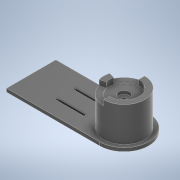
# Autodesk Inventor part: Base
Saved by Autodesk Inventor 2022.3 (Build 263350000, 350)
## iProperties
Created: 2022-05-27
Part Number: Base
Material: PC/ABS Plastic
Document SubType Name: Modeling
Designer: Mlees
Density: 0.357273 g/cm^3
Appearance: Smooth - White
Author: Mlees
Autodesk Inventor part; units mm, degrees
ref_plane "YZ Plane" through (0, 0, 0) normal (1, 0, 0) x (0, 1, 0)
ref_plane "XZ Plane" through (0, 0, 0) normal (0, 1, 0) x (-1, 0, 0)
ref_plane "XY Plane" through (0, 0, 0) normal (0, 0, 1) x (1, 0, 0)
sketch "Sketch1" plane through (0, 0, 0) normal (0, 1, 0) x (-1, 0, 0)
  line L0 (-100, 300) -> (100, 300)
  line L1 (100, 300) -> (100, -100)
  line L2 (100, -100) -> (-100, -100)
  line L3 (-100, -100) -> (-100, 300)
  point P0 (0, 0)
  dimension "d4" = 200
  dimension "d5" = 400
  constraints: 8 end point, 2 parallel, 1 horizontal, 1 perpendicular
  measures "d4" distance of L1.end L2.end
  measures "d5" distance of L0.end L1.end
extrude "Extrusion1" add sketch "Sketch1" along normal blind 5
sketch "Sketch2" plane through (0, 5, 0) normal (0, 1, 0) x (1, 0, 0)
  circle A0 centre (0, 0) radius 3
  circle A1 centre (0, 0) radius 30
  dimension "d10" = 6
  dimension "d11" = 60
  constraints: 2 centre point, 2 coincident
  measures "d10" diameter of A0
  measures "d11" diameter of A1
extrude "Extrusion2" add sketch "Sketch2" along normal blind 41.5
sketch "Sketch3" plane through (0, 46.5, 0) normal (0, 1, 0) x (1, 0, 0)
  circle A0 centre (0, 0) radius 3 projected
  circle A1 centre (0, 0) radius 30
  circle A2 centre (0, 0) radius 21.5
  circle A3 centre (0, 0) radius 3
  dimension "d14" = 43
  dimension "d15" = 6
  constraints: 3 centre point, 3 coincident
  measures "d14" diameter of A2
  measures "d15" diameter of A3
extrude "Extrusion3" add sketch "Sketch3" along normal blind 1 contours A1
sketch "Sketch4" plane through (0, 47.5, 0) normal (0, 1, 0) x (1, 0, 0)
  circle A0 centre (0, 0) radius 21.5 projected
  line L0 (-21.5, 0) -> (-30, 0)
  circle A1 centre (0, 0) radius 30 projected
  line L1 (21.633, 0) -> (30.1771, 0)
  circle A2 centre (0, 0) radius 3 projected
  arc A3 (21.633, 0) -> (-21.633, 0) centre (0, 0) ccw
  point P0 (30, 0)
  constraints: 4 end point, 3 point on line, 2 point on circle, 1 centre point, 1 coincident, 1 horizontal, 1 horizontal alignment, 3 other
extrude "Extrusion4" add sketch "Sketch4" along normal blind 15 contours L0 A1 L1 A3 picked at (-26.7109, 4.1189)
sketch "Sketch5" plane through (0, 5, 0) normal (0, 1, 0) x (1, 0, 0)
  line L0 (-13, 0) -> (13, 0)
  arc A0 (-11.5, -45) -> (-14.5, -45) centre (-13, -45) ccw
  line L1 (-14.5, -45) -> (-14.5, -85)
  arc A1 (-14.5, -85) -> (-11.5, -85) centre (-13, -85) ccw
  line L2 (-11.5, -45) -> (-11.5, -85)
  line L3 (0, 0) -> (0, -51.7204)
  arc A2 (14.5, -45) -> (11.5, -45) centre (13, -45) ccw
  line L4 (14.5, -45) -> (14.5, -85)
  arc A3 (11.5, -85) -> (14.5, -85) centre (13, -85) ccw
  line L5 (11.5, -45) -> (11.5, -85)
  dimension "d20" = 13
  dimension "d21" = 26
  dimension "d22" = 45
  dimension "d24" = 40
  constraints: 12 end point, 8 point on circle, 5 symmetric about line, 4 centre point, 2 tangent, 2 vertical, 2 other
  measures "d20" distance of L3.start L0.start
  measures "d21" distance of L0.start L0.end
  measures "d22" distance of L0.end A2.centre
  measures "d24" distance of L1.start L1.end
extrude "Extrusion5" cut sketch "Sketch5" against normal through all
fillet "Fillet1" radius 2 8 edges at (13, 0, 43.5) (11.5, 0, 65) (13, 0, 86.5) (14.5, 0, 65) (-13, 0, 43.5) (-14.5, 0, 65) (-13, 0, 86.5) (-11.5, 0, 65) inverted yes
sketch "Sketch6" plane through (0, 47.5, 0) normal (0, 1, 0) x (1, 0, 0)
  circle A0 centre (0, 0) radius 3 projected
  circle A1 centre (0, 0) radius 30
  circle A2 centre (0, 0) radius 21.5
  circle A3 centre (0, 0) radius 30 projected
  line L0 (0, 0) -> (30, 0) construction
  line L1 (0, 0) -> (30, 0) construction
  line L2 (-5.5646, -20.7674) -> (-7.7646, -28.9778)
  line L3 (5.5646, -20.7674) -> (7.7646, -28.9778)
  constraints: 8 end point, 4 point on circle, 2 centre point, 2 coincident, 2 horizontal
extrude "Extrusion6" add sketch "Sketch6" along normal up to surface (15 mm away) contours L2 A2 L3 A1 picked at (5.3146, -26.5437)
sketch "Sketch7" plane through (0, 5, 0) normal (0, 1, 0) x (1, 0, 0)
  circle A0 centre (0, 0) radius 3 projected
  line L0 (-50, 0) -> (-50, 50)
  line L1 (-50, 50) -> (50, 50)
  line L2 (50, 50) -> (50, -150)
  line L3 (50, -150) -> (-50, -150)
  line L4 (-50, -150) -> (-50, 0)
  line L5 (-100, 100) -> (-100, -300) projected
  line L6 (-100, -300) -> (100, -300)
  line L7 (100, -300) -> (100, 100)
  line L8 (100, 100) -> (-100, 100)
  line L9 (-100, 100) -> (-100, -300)
  dimension "d32" = 50
  dimension "d33" = 50
  dimension "d34" = 100
  dimension "d35" = 200
  constraints: 18 end point, 4 perpendicular, 2 parallel, 1 collinear, 1 horizontal, 1 point on line, 1 vertical
  measures "d32" distance of A0.centre L0.start
  measures "d33" distance of L0.start L0.end
  measures "d34" distance of L0.end L1.end
  measures "d35" distance of L1.end L2.end
extrude "Extrusion7" cut sketch "Sketch7" against normal through all contours L8 L7 L6 L5
sketch "Sketch8" plane through (0, 62.5, 0) normal (0, 1, 0) x (1, 0, 0)
  circle A0 centre (0, 0) radius 3 projected
  arc A1 (-7.7646, -28.9778) -> (7.7646, -28.9778) centre (0, 0) ccw projected
  circle A2 centre (0, 0) radius 30
  line L0 (-7.7646, -28.9778) -> (-5.5646, -20.7674) projected
  circle A3 centre (0, 0) radius 21.5
  line L1 (-5.5646, -20.7674) -> (-7.7646, -28.9778)
  line L2 (5.5646, -20.7674) -> (7.7646, -28.9778) projected
  line L3 (5.5646, -20.7674) -> (7.7646, -28.9778)
  arc A4 (21.633, 0) -> (-21.633, 0) centre (0, 0) ccw projected
  line L4 (-21.633, 0) -> (-30, 0) projected
  line L5 (-21.633, 0) -> (-30, 0)
  line L6 (21.633, 0) -> (30, 0) projected
  arc A5 (30, 0) -> (-30, 0) centre (0, 0) ccw projected
  line L7 (21.633, 0) -> (30, 0)
  constraints: 8 end point, 2 centre point, 2 coincident, 2 collinear, 2 horizontal, 2 point on circle
extrude "Extrusion8" cut sketch "Sketch8" against normal blind 7 contours L0 A3 L2 A1 | A2 L6 A4 L4
sketch "Sketch10" plane through (0, 46.5, 0) normal (0, 1, 0) x (1, 0, 0)
  circle A0 centre (0, 0) radius 8.125
  constraints: 1 centre point, 1 coincident
extrude "Extrusion10" cut sketch "Sketch10" against normal blind 5
sketch "Sketch11" plane through (-50, 5, 150) normal (0, 0, 1) x (1, 0, 0)
  line L0 (100, 0) -> (100, -5) projected
  line L1 (0, -5) -> (100, -5)
  line L2 (100, -5) -> (100, 0)
  line L3 (100, 0) -> (0, 0)
  line L4 (0, 0) -> (0, -5)
  point P0 (50, -5)
  constraints: 8 end point, 2 parallel, 1 horizontal, 1 perpendicular
extrude "Extrusion11" cut sketch "Sketch11" against normal blind 14
sketch "Sketch12" plane through (0, 5, 0) normal (0, 1, 0) x (1, 0, 0)
  arc A0 (36, 0) -> (-36, 0) centre (0, 0) ccw
  line L0 (36, 0) -> (36, -136)
  line L1 (50, -136) -> (-50, -136) projected
  line L2 (50, 50) -> (50, -136) projected
  line L3 (36, -136) -> (50, -136)
  line L4 (50, -136) -> (50, 50)
  line L5 (50, 50) -> (-50, 50)
  line L6 (-50, -136) -> (-50, 50) projected
  line L7 (-50, 50) -> (-50, -136)
  line L8 (-50, -136) -> (-36, -136)
  line L9 (-36, -136) -> (-36, 0)
  dimension "d47" = 72
  constraints: 14 end point, 2 collinear, 2 perpendicular, 2 point on circle, 2 point on line, 1 centre point, 1 coincident, 1 tangent, 1 vertical
  measures "d47" diameter of A0
extrude "Extrusion12" cut sketch "Sketch12" against normal through all contours A0 L9 L1 L6 L5 L2 L0
sketch "Sketch13" plane through (0, 0, 0) normal (0, -1, 0) x (1, 0, 0)
  circle A0 centre (0, 0) radius 3 projected
  line L0 (0, -12.5) -> (12.5, -12.5)
  line L1 (12.5, -12.5) -> (-12.5, -12.5)
  line L2 (-12.5, -12.5) -> (-12.5, 12.5)
  line L3 (-12.5, 12.5) -> (12.5, 12.5)
  line L4 (12.5, 12.5) -> (12.5, -12.5)
  dimension "d50" = 12.5
  dimension "d51" = 12.5
  dimension "d52" = 25
  dimension "d53" = 25
  constraints: 10 end point, 2 parallel, 1 horizontal, 1 perpendicular
  measures "d50" distance of A0.centre L0.start
  measures "d51" distance of L0.start L0.end
  measures "d52" distance of L2.end L3.end
  measures "d53" distance of L1.end L2.end
extrude "Extrusion13" cut sketch "Sketch13" against normal blind 12.5 contours A0 | L1 L2 L3 L4 L0
sketch "Sketch14" plane through (0, 0, 0) normal (0, -1, 0) x (1, 0, 0)
  line L0 (-12.5, 12.5) -> (12.5, 12.5) projected
  line L1 (12.5, 12.5) -> (-12.5, 12.5)
  line L2 (-12.5, 12.5) -> (-12.5, 18.5)
  line L3 (-12.5, 18.5) -> (12.5, 18.5)
  line L4 (12.5, 18.5) -> (12.5, 12.5)
  line L5 (12.5, 12.5) -> (12.5, -12.5) projected
  line L6 (12.5, -12.5) -> (-12.5, -12.5)
  line L7 (-12.5, -12.5) -> (-12.5, -18.5)
  line L8 (-12.5, -18.5) -> (12.5, -18.5)
  line L9 (12.5, -18.5) -> (12.5, -12.5)
  point P0 (0, 0)
  dimension "d56" = 6
  dimension "d57" = 25
  dimension "d58" = 6
  constraints: 16 end point, 4 parallel, 2 horizontal, 2 perpendicular
  measures "d56" distance of L1.end L2.end
  measures "d57" distance of L8.end L7.end
  measures "d58" distance of L7.end L6.end
extrude "Extrusion14" cut sketch "Sketch14" against normal blind 2
sketch "Sketch15" plane through (0, 2, 0) normal (0, -1, 0) x (1, 0, 0)
  line L0 (12.5, 18.5) -> (12.5, 12.5) projected
  line L1 (-12.5, -18.5) -> (-12.5, 18.5) projected
  circle A0 centre (-7.5, 15.5) radius 1.5
  circle A1 centre (7.5, 15.5) radius 1.5
  line L2 (12.5, 12.5) -> (12.5, -12.5) projected
  circle A2 centre (-7.5, -15.5) radius 1.5
  circle A3 centre (7.5, -15.5) radius 1.5
  point P0 (0, 0)
  dimension "d64" = 3
  constraints: 4 centre point
  measures "d64" diameter of A0
extrude "Extrusion15" cut sketch "Sketch15" against normal blind 5
ref_plane "Work Plane1" through (12.5, 12.5, 0) normal (0, 0, -1) x (-1, 0, 0)
sketch "Sketch16" plane through (12.5, 12.5, 12.5) normal (0, 0, -1) x (-1, 0, 0)
  line L0 (0, -10.5) -> (25, -10.5) projected
  circle A0 centre (12.5, -3.5) radius 3
  point P0 (12.5, -12.5)
  dimension "d68" = 6
  constraints: 1 centre point
  measures "d68" diameter of A0
sketch "Sketch17" plane through (36, 5, 136) normal (1, 0, 0) x (0, 0, -1)
  line L0 (123.5, -3) -> (123.5, 7.5) projected
  line L1 (123.5, 4.0615) -> (105.3233, 4.0615)
  point P0 (136, -5)
  constraints: 2 end point, 1 horizontal, 1 point on line
sweep "Sweep1" cut profiles "Sketch16" path "Sketch17" path curves L1
sketch "Sketch18" plane through (0, 12.5, 0) normal (0, -1, 0) x (1, 0, 0)
  circle A0 centre (0, 0) radius 6
  dimension "d71" = 12
  constraints: 1 centre point, 1 coincident
  measures "d71" diameter of A0
extrude "Extrusion16" cut sketch "Sketch18" against normal blind 5
body "Solid1"
